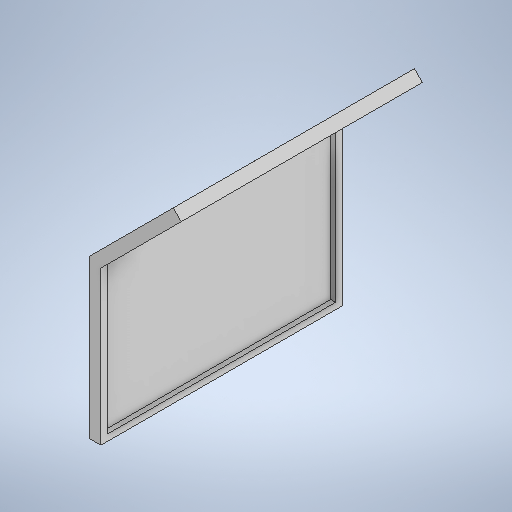
# Autodesk Inventor part: lid
Saved by Autodesk Inventor 2026.1 (Build 301233000, 233)
## iProperties
Created: 2026-08-16
Part Number: lid
Material: Generic
Document SubType Name: Modeling
Designer: rowan
Density: 1 g/cm^3
Appearance: Default
Author: rowan
Autodesk Inventor part; units mm, degrees
ref_plane "YZ Plane" through (0, 0, 0) normal (1, 0, 0) x (0, 1, 0)
ref_plane "XZ Plane" through (0, 0, 0) normal (0, 1, 0) x (-1, 0, 0)
ref_plane "XY Plane" through (0, 0, 0) normal (0, 0, 1) x (1, 0, 0)
sketch "Sketch1" plane through (0, 0, 0) normal (0, 1, 0) x (-1, 0, 0)
  line L0 (0, 0) -> (7, 0)
  line L1 (7, 0) -> (7, -150)
  line L2 (7, -150) -> (0, -150)
  line L3 (0, -150) -> (0, -146)
  line L4 (0, -146) -> (3, -146)
  line L5 (3, -146) -> (3, -4)
  line L6 (3, -4) -> (0, -4)
  line L7 (0, -4) -> (0, 0)
  dimension "d4" = 7
  dimension "d5" = 3
  dimension "d6" = 4
  dimension "d7" = 150
  constraints: 16 end point, 7 perpendicular, 1 collinear, 1 horizontal, 1 point on line
  measures "d4" distance of L1.end L2.end
  measures "d5" distance of L3.end L4.end
  measures "d6" distance of L2.end L3.end
  measures "d7" distance of L0.end L1.end
sketch "Sketch2" plane through (0, 0, 0) normal (0, 0, 1) x (1, 0, 0)
  line L0 (0, 0) -> (0, 95.438)
  line L1 (0, 95.438) -> (49.962, 145.4)
  dimension "d8" = 135
  dimension "d9" = 95.438
  dimension "d10" = 70.657
  constraints: 4 end point, 1 vertical
  measures "d8" angle of L0 L1
  measures "d9" distance of L0.start L0.end
  measures "d10" distance of L0.end L1.end
sweep "Sweep1" add profiles "Sketch1" path "Sketch2"
sketch "Sketch3" plane through (45.0123, 150.3498, -150) normal (0.7071, 0.7071, 0) x (-0.7071, 0.7071, 0)
  line L0 (-7, 150) -> (-7, 146) projected
  line L1 (-74.4849, 4) -> (-7, 4) projected
  line L2 (-7, 146) -> (-7, 4)
  line L3 (-72.3635, 146) -> (-4, 146) projected
  line L4 (-7, 146) -> (-4, 146)
  line L5 (-4, 4) -> (-7, 4) projected
  line L6 (-4, 146) -> (-4, 4)
  line L7 (-4, 4) -> (-7, 4)
  point P0 (-74.4849, 150)
  constraints: 8 end point, 2 collinear, 2 perpendicular
extrude "Extrusion1" add sketch "Sketch3" against normal blind 5.657
sketch "Sketch5" plane through (-7, 0, 0) normal (0, -1, 0) x (1, 0, 0)
  line L0 (4, -4) -> (4, -146) projected
  line L1 (7, -4) -> (4, -4) projected
  line L2 (4, -146) -> (7, -146) projected
  line L3 (7, -146) -> (7, -4)
  line L4 (7, -146) -> (7, -150) projected
  point P0 (7, 0)
  constraints: 2 end point, 1 collinear
extrude "Extrusion2" add sketch "Sketch5" against normal blind 4
sketch "Sketch6" plane through (-7, 98.3375, -150) normal (-0.7071, 0.7071, 0) x (-0.7071, -0.7071, 0)
  line L0 (-16.7782, 123.5) -> (-56.7782, 123.5)
  line L1 (-56.7782, 123.5) -> (-56.7782, 26.5)
  line L2 (-56.7782, 26.5) -> (-16.7782, 26.5)
  line L3 (-16.7782, 26.5) -> (-16.7782, 123.5)
  line L4 (0, 0) -> (0, 150) projected
  line L5 (0, 0) -> (-73.5565, 0) projected
  point P0 (64.5854, 150)
  point P1 (-16.7782, 75)
  point P2 (0, 75)
  point P3 (-36.7782, 26.5)
  point P4 (-36.7782, 0)
  dimension "d17" = 97
  dimension "d18" = 40
  constraints: 8 end point, 4 midpoint, 2 parallel, 1 horizontal, 1 horizontal alignment, 1 perpendicular, 1 vertical alignment
  measures "d17" distance of L2.end L0.start
  measures "d18" distance of L0.start L0.end
extrude "Extrusion3" cut sketch "Sketch6" against normal blind 4
body "Solid1"
